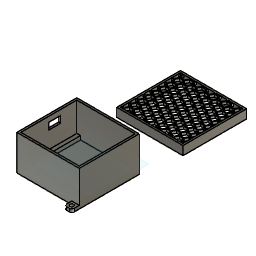
arduino_imu case_ (Autodesk Fusion 360 design; units mm, degrees)
Autodesk Fusion 360 part; units mm, degrees
(part 1 of 2)
sketch "Sketch1" plane through (0, 0, 0) normal (0, 0, 1) x (1, 0, 0)
sketch "Sketch2" plane through (0, 0, 0) normal (0, 0, 1) x (1, 0, 0)
  line L0 (0, 0) -> (46.5, 0)
  line L1 (46.5, 0) -> (46.5, 44.5)
  line L2 (46.5, 44.5) -> (0, 44.5)
  line L3 (0, 44.5) -> (0, 0)
  dimension "d1" = 46.5
  dimension "d2" = 44.5
  constraint horizontal L0
  constraint vertical L1
  constraint horizontal L2
  constraint vertical L3
  constraint coincident L0.start L3.end
  measures "d1" distance of L0.start L0.end
  measures "d2" distance of L0.start L2.end
extrude "Extrude1" add sketch "Sketch2" along normal blind 2 makes body 1
sketch "Sketch3" plane through (0, 0, 2) normal (0, 0, 1) x (-1, 0, 0)
  line L0 (0, -44.5) -> (0, 0)
  line L1 (0, 0) -> (-46.5, 0)
  line L2 (-46.5, 0) -> (-46.5, -44.5)
  line L3 (-46.5, -44.5) -> (0, -44.5)
sketch "Sketch4" plane through (0, 0, 2) normal (0, 0, 1) x (-1, 0, 0)
  line L0 (0, -44.5) -> (0, 0)
  line L1 (0, 0) -> (-46.5, 0)
  line L2 (-46.5, 0) -> (-46.5, -44.5)
  line L3 (-46.5, -44.5) -> (0, -44.5)
  line L4 (1.6, 1.6) -> (-48.1, 1.6)
  line L5 (-48.1, 1.6) -> (-48.1, -46.1)
  line L6 (-48.1, -46.1) -> (1.6, -46.1)
  line L7 (1.6, -46.1) -> (1.6, 1.6)
  dimension "d5" = 1.6
extrude "Extrude2" add sketch "Sketch4" against normal blind 22 bodies 1
copy_body "Body->Comp1" bodies 1 removing the originals makes body 2 in component "Component"
sketch "Sketch5" plane through (0, 0, 2.4305) normal (0, 0, 1) x (-1, 0, 0)
  line L0 (0, -33.8) -> (0, 10.7)
  line L1 (0, 10.7) -> (-46.5, 10.7)
  line L2 (-46.5, 10.7) -> (-46.5, -33.8)
  line L3 (-46.5, -33.8) -> (0, -33.8)
  line L4 (0, -33.8) -> (-3, -33.8)
  line L5 (-3, -33.8) -> (-3, 10.7)
  line L6 (-3, 10.7) -> (0, 10.7)
  line L7 (0, 10.7) -> (0, -33.8)
  line L8 (-46.5, -33.8) -> (-43.5, -33.8)
  line L9 (-43.5, -33.8) -> (-43.5, 10.7)
  line L10 (-43.5, 10.7) -> (-46.5, 10.7)
  line L11 (-46.5, 10.7) -> (-46.5, -33.8)
  dimension "d8" = 3
  dimension "d9" = 3
  constraint horizontal L4
  constraint vertical L5
  constraint horizontal L6
  constraint vertical L7
  constraint coincident L1 L5.end
  constraint coincident L0.start L3.end
  constraint horizontal L8
  constraint vertical L9
  constraint horizontal L10
  constraint vertical L11
  constraint coincident L1 L9.end
  constraint coincident L2.end L3.start
  measures "d8" distance of L0.start L4.end
  measures "d9" distance of L2.end L8.end
extrude "Extrude1'" add sketch "Sketch5" along normal blind 3 contours L0 L1 L3 L4 L5 L6 L7 | L1 L2 L3 L8 L9 L10 L11 sketch seen with x (1, 0, 0) y (0, -1, 0) z (0, 0, -1) at (0, 33.8, 2.4305) bodies 2 in component "Component"
sketch "Sketch6" plane through (0, 0, 0) normal (1, 0, 0) x (0, 1, 0)
  line L0 (-10.7, 5.4305) -> (33.8, 5.4305)
  line L1 (33.8, 5.4305) -> (33.8, 22.4305)
  line L2 (33.8, 22.4305) -> (-10.7, 22.4305)
  line L3 (-10.7, 22.4305) -> (-10.7, 5.4305)
  line L4 (11.55, 5.4305) -> (11.55, 20.4305)
  line L5 (16.55, 17.9305) -> (6.55, 17.9305)
  line L6 (6.55, 17.9305) -> (6.55, 22.9305)
  line L7 (6.55, 22.9305) -> (16.55, 22.9305)
  line L8 (16.55, 22.9305) -> (16.55, 17.9305)
  line L9 (16.55, 17.9305) -> (6.55, 22.9305) construction
  line L10 (6.55, 17.9305) -> (16.55, 22.9305) construction
  point P0 (11.55, 20.4305)
  dimension "d12" = 15
  dimension "d13" = 10
  dimension "d14" = 5
  constraint midpoint L0 L4.start
  constraint perpendicular L0 L4
  constraint horizontal L5
  constraint perpendicular L5 L6
  constraint parallel L5 L7
  constraint parallel L6 L8
  constraint coincident L9 P0
  constraint coincident L10 P0
  constraint coincident P0 L4.end
  measures "d12" distance of L4.start P0
  measures "d13" distance of L6.end L7.end
  measures "d14" distance of L5.end L6.end
extrude "Extrude2'" add 1 faces at (31, 45.5667, -20) along direction (0, 0, -1) blind 2 on bodies 2 bodies 2 in component "Component"
extrude "Extrude3" cut sketch "Sketch6" against normal blind 2.5 contours L2 L5 L6 L8 | L2 L6 L7 L8 sketch seen with x (1, 0, 0) y (0, -1, 0) z (0, 0, -1) at (0, 33.8, 2.4305) bodies 2 in component "Component"
sketch "Sketch7" plane through (0, 0, 24.4305) normal (0, 0, 1) x (-1, 0, 0)
  line L0 (-46.5, 10.7) -> (0, 10.7)
  line L1 (0, 10.7) -> (0, -33.8)
  line L2 (0, -33.8) -> (-46.5, -33.8)
  line L3 (-46.5, -33.8) -> (-46.5, 10.7)
  line L4 (1.6, -35.4) -> (1.6, 12.3)
  line L5 (1.6, 12.3) -> (-48.1, 12.3)
  line L6 (-48.1, 12.3) -> (-48.1, -35.4)
  line L7 (-48.1, -35.4) -> (1.6, -35.4)
  line L8 (0, 10.7) -> (-46.5, 10.7)
  line L9 (-46.5, 10.7) -> (-46.5, -33.8)
  line L10 (-46.5, -33.8) -> (0, -33.8)
  line L11 (0, -33.8) -> (0, 10.7)
  line L12 (0, -33.8) -> (-46.5, -33.8)
  line L13 (0, 10.7) -> (0, -33.8)
  line L14 (-46.5, 10.7) -> (0, 10.7)
  line L15 (-46.5, -33.8) -> (-46.5, 10.7)
  line L16 (-1, 9.7) -> (-45.5, 9.7)
  line L17 (-45.5, 9.7) -> (-45.5, -32.8)
  line L18 (-45.5, -32.8) -> (-1, -32.8)
  line L19 (-1, -32.8) -> (-1, 9.7)
  dimension "d19" = -1
  constraint horizontal L8
  constraint vertical L9
  constraint horizontal L10
  constraint vertical L11
  constraint coincident L2.end L3.start
  constraint coincident L0.end L1.start
extrude "Extrude1''" add sketch "Sketch7" against normal blind 3 separate body contours L0 L1 L2 L3 L8 L9 L10 L11 L12 L13 L14 L15 makes body 3 in component "Component'"
sketch "Sketch8" plane through (0, 0, 24.4305) normal (0, 0, 1) x (-1, 0, 0)
  line L0 (-1, 9.7) -> (-1, -32.8)
  line L1 (-1, -32.8) -> (-45.5, -32.8)
  line L2 (-45.5, -32.8) -> (-45.5, 9.7)
  line L3 (-45.5, 9.7) -> (-1, 9.7)
  line L4 (-46.5, -33.8) -> (0, -33.8)
  line L5 (0, -33.8) -> (0, 10.7)
  line L6 (0, 10.7) -> (-46.5, 10.7)
  line L7 (-46.5, 10.7) -> (-46.5, -33.8)
  line L8 (1, 1) -> (-48, 1)
  line L9 (-48, 1) -> (-48, -35)
  line L10 (-48, -35) -> (1, -35)
  line L11 (1, -35) -> (1, 1)
  constraint horizontal L8
  constraint vertical L9
  constraint horizontal L10
  constraint vertical L11
extrude "Extrude2''" add sketch "Sketch8" along normal blind 1.5 contours L0 L1 L2 L4 L5 L7 L8 | L0 L1 L2 L8 | L4 L5 L7 L8 L9 L10 L11 bodies 3 in component "Component'"
move_body "Move1" bodies 3 to x (1, 0, 0) y (0, -1, 0) z (0, 0, -1) at (-0.0377, 29.218, 33.0505) in component "Component'"
sketch "Sketch9" plane through (0, 0, 2.2652) normal (0, 0, 1) x (-1, 0, 0)
  line L0 (-2.9332, -33.7586) -> (-2.9332, 10.7414)
  line L1 (-2.9332, 10.7414) -> (-43.4332, 10.7414)
  line L2 (-43.4332, 10.7414) -> (-43.4332, -33.7586)
  line L3 (-43.4332, -33.7586) -> (-2.9332, -33.7586)
sketch "Sketch10" plane through (0, 0, 2.2652) normal (0, 0, 1) x (-1, 0, 0)
  line L0 (-43.4332, -33.7586) -> (-2.9332, -33.7586)
  line L1 (-2.9332, -33.7586) -> (-2.9332, 10.7414)
  circle A0 centre (-14.9332, 8.7414) radius 2.5
  point P0 (-14.9332, 8.7414)
  dimension "d24" = 42.5
  dimension "d25" = 12
  dimension "d52" = 5
  constraint coincident P0 A0.centre
  measures "d24" distance of P0 L0
  measures "d25" distance of P0 L1
  measures "d52" diameter of A0
extrude "Extrude4" add sketch "Sketch10" along normal blind 17 sketch seen with x (1, 0, 0) y (0, -1, 0) z (0, 0, -1) at (0.0668, 33.7586, 2.2652) bodies 2 in component "Component"
hole "Hole1" at (15.0254, 42.4284, -17) direction (0, 0, 1) diameter 3.1 depth 6 tip angle 118 bodies 2 in component "Component"
extrude "Extrude5" cut 1 faces at (-1.0667, 17.25, -17.1667) along direction (0, -1, 0) blind 5 on bodies 2 bodies 2 in component "Component"
extrude "Extrude6" add 1 faces at (-0.5333, 27.25, -17.1667) along direction (0, -1, 0) blind 5 on bodies 2 bodies 2 in component "Component"
extrude "Extrude7" add 1 faces at (31, 45.5667, -22) along direction (0, 0, -1) blind 2 on bodies 2 bodies 2 in component "Component"
extrude "Extrude8" add 1 faces at (-1.0667, 15.5833, -15.5) along direction (0, 0, -1) blind 2 on bodies 2 bodies 2 in component "Component"
extrude "Extrude9" cut 1 faces at (-1.0667, 15.5833, -20.5) along direction (0, 0, -1) blind 2.3 on bodies 2 bodies 2 in component "Component"
sketch "Sketch11" plane through (0, 0, 5.2652) normal (0, 0, 1) x (-1, 0, 0)
  line L0 (-46.4332, 10.7414) -> (-46.4332, -33.7586)
  line L1 (-46.4332, -33.7586) -> (-43.4332, -33.7586)
  line L2 (-43.4332, -33.7586) -> (-43.4332, 10.7414)
  line L3 (-43.4332, 10.7414) -> (-46.4332, 10.7414)
  line L4 (-46.4332, -0.2586) -> (-43.4332, -0.2586)
  line L5 (-43.4332, -0.2586) -> (-43.4332, 1.4358)
  line L6 (-43.4332, 1.4358) -> (-46.4332, 1.4358)
  line L7 (-46.4332, 1.4358) -> (-46.4332, -0.2586)
  dimension "d41" = 33.5
  constraint horizontal L4
  constraint vertical L5
  constraint horizontal L6
  constraint vertical L7
  constraint coincident L2 L5.end
  constraint coincident L0 L4.start
  measures "d41" distance of L1 L4
extrude "Extrude10" add sketch "Sketch11" along normal blind 2 contours L0 L2 L4 L5 L6 L7 sketch seen with x (1, 0, 0) y (0, -1, 0) z (0, 0, -1) at (0.0668, 33.7586, 2.2652) bodies 2 in component "Component"
ref_plane "WorkPlane1" through (23.1832, 11.5086, 13.2652) normal (1, 0, 0) x (0, 1, 0)
mirror "Mirror1" about plane through (23.25, 22.25, -11) normal (1, 0, 0) of "Extrude10" in component "Component"
extrude "Extrude11" add 1 faces at (-1.0667, 15.5833, -22.8) along direction (0, 0, 1) blind 1 on bodies 2 bodies 2 in component "Component"
extrude "Extrude12" cut 1 faces at (-1.0667, 15.5833, -17.5) along direction (0, 0, 1) blind 1 on bodies 2 bodies 2 in component "Component"
extrude "Extrude13" add 1 faces at (-1.0667, 12.25, -18.2667) along direction (0, 1, 0) blind 0.5 on bodies 2 bodies 2 in component "Component"
extrude "Extrude14" add 1 faces at (31, 45.5667, -24) along direction (0, 0, -1) blind 2 on bodies 2 bodies 2 in component "Component"
sketch "Sketch12" plane through (0, -12.3414, 0) normal (0, -1, 0) x (1, 0, 0)
  line L0 (-1.6668, 0.2652) -> (48.0332, 0.2652)
  line L1 (48.0332, 0.2652) -> (48.0332, 28.2652)
  line L2 (48.0332, 28.2652) -> (-1.6668, 28.2652)
  line L3 (-1.6668, 28.2652) -> (-1.6668, 0.2652)
  line L4 (48.0332, 0.2652) -> (42.0332, 0.2652)
  line L5 (42.0332, 0.2652) -> (42.0332, 2.7652)
  line L6 (42.0332, 2.7652) -> (48.0332, 2.7652)
  line L7 (48.0332, 2.7652) -> (48.0332, 0.2652)
  dimension "d55" = 6
  dimension "d56" = 2.5
  constraint horizontal L4
  constraint vertical L5
  constraint horizontal L6
  constraint vertical L7
  constraint coincident L0.end L1.start
  measures "d55" distance of L0.end L4.end
  measures "d56" distance of L0.end L6.end
extrude "Extrude15" add sketch "Sketch12" along normal blind 6 contours L0 L1 L4 L5 L6 L7 sketch seen with x (1, 0, 0) y (0, -1, 0) z (0, 0, -1) at (0.0668, 33.7586, 2.2652) bodies 2 in component "Component"
hole "Hole2" at (45.1, 49.1, -0.5) direction (0, 0, 1) diameter 3 depth 7 tip angle 118 bodies 2 in component "Component"
sketch "Sketch13" plane through (0, 35.3586, 0) normal (0, 1, 0) x (-1, 0, 0)
  line L0 (-48.0332, 0.2652) -> (1.6668, 0.2652)
  line L1 (1.6668, 0.2652) -> (1.6668, 28.2652)
  line L2 (1.6668, 28.2652) -> (-48.0332, 28.2652)
  line L3 (-48.0332, 28.2652) -> (-48.0332, 0.2652)
  line L4 (1.6668, 0.2652) -> (-4.3332, 0.2652)
  line L5 (-4.3332, 0.2652) -> (-4.3332, 2.7652)
  line L6 (-4.3332, 2.7652) -> (1.6668, 2.7652)
  line L7 (1.6668, 2.7652) -> (1.6668, 0.2652)
  dimension "d62" = 6
  dimension "d63" = 2.5
  constraint horizontal L4
  constraint vertical L5
  constraint horizontal L6
  constraint vertical L7
  constraint coincident L0.end L1.start
  measures "d62" distance of L0.end L4.end
  measures "d63" distance of L0.end L6.end
extrude "Extrude16" add sketch "Sketch13" along normal blind 6 contours L0 L1 L4 L5 L6 L7 sketch seen with x (1, 0, 0) y (0, -1, 0) z (0, 0, -1) at (0.0668, 33.7586, 2.2652) bodies 2 in component "Component"
hole "Hole3" at (1.4, -4.6, -0.5) direction (0, 0, 1) diameter 3 depth 7 tip angle 118 bodies 2 in component "Component"
fillet "Fillet1" radius 2 4 edges at (48.1, 52.1, 0.75) (42.1, 52.1, 0.75) (4.4, -7.6, 0.75) (-1.6, -7.6, 0.75) on bodies 2 in component "Component"
sketch "Sketch14" plane through (0, 0, 28.2652) normal (0, 0, 1) x (-1, 0, 0)
  line L0 (-46.4332, 10.7414) -> (0.0668, 10.7414)
  line L1 (0.0668, 10.7414) -> (0.0668, -33.7586)
  line L2 (0.0668, -33.7586) -> (-46.4332, -33.7586)
  line L3 (-46.4332, -33.7586) -> (-46.4332, 10.7414)
  line L4 (1.6668, -35.3586) -> (1.6668, 12.3414)
  line L5 (1.6668, 12.3414) -> (-48.0332, 12.3414)
  line L6 (-48.0332, 12.3414) -> (-48.0332, -35.3586)
  line L7 (-48.0332, -35.3586) -> (1.6668, -35.3586)
  line L8 (-49.5332, -36.8586) -> (3.1668, -36.8586)
  line L9 (3.1668, -36.8586) -> (3.1668, 13.8414)
  line L10 (3.1668, 13.8414) -> (-49.5332, 13.8414)
  line L11 (-49.5332, 13.8414) -> (-49.5332, -36.8586)
  dimension "d71" = 1.5
extrude "Extrude1'''" add sketch "Sketch14" against normal blind 4 separate body contours L8 L9 L10 L11 makes body 4 in component "Component''"
sketch "Sketch15" plane through (0, 0, 28.2652) normal (0, 0, 1) x (-1, 0, 0)
  line L0 (1.6668, -35.3586) -> (-48.0332, -35.3586)
  line L1 (-48.0332, -35.3586) -> (-48.0332, 12.3414)
  line L2 (-48.0332, 12.3414) -> (1.6668, 12.3414)
  line L3 (1.6668, 12.3414) -> (1.6668, -35.3586)
  line L4 (-49.5332, 13.8414) -> (-49.5332, -36.8586)
  line L5 (-49.5332, -36.8586) -> (3.1668, -36.8586)
  line L6 (3.1668, -36.8586) -> (3.1668, 13.8414)
  line L7 (3.1668, 13.8414) -> (-49.5332, 13.8414)
extrude "Extrude2'''" add sketch "Sketch15" along normal blind 2 contours L0 L1 L2 L3 | L4 L5 L6 L7 bodies 4 in component "Component''"
sketch "Sketch16" plane through (0, 0, 6.5217) normal (0, 0, -1) x (1, 0, 0)
  line L0 (51.3034, -114.6661) -> (51.3034, -66.9661)
  line L1 (51.3034, -66.9661) -> (1.6034, -66.9661)
  line L2 (1.6034, -66.9661) -> (1.6034, -114.6661)
  line L3 (1.6034, -114.6661) -> (51.3034, -114.6661)
  line L4 (51.3034, -90.8161) -> (1.6034, -90.8161)
  line L5 (26.4534, -114.6661) -> (26.4534, -90.8161)
  line L6 (27.8967, -93.3161) -> (29.3401, -90.8161)
  line L7 (29.3401, -90.8161) -> (27.8967, -88.3161)
  line L8 (27.8967, -88.3161) -> (25.01, -88.3161)
  line L9 (25.01, -88.3161) -> (23.5666, -90.8161)
  line L10 (23.5666, -90.8161) -> (25.01, -93.3161)
  line L11 (25.01, -93.3161) -> (27.8967, -93.3161)
  line L12 (28.6184, -89.5661) -> (26.4534, -90.8161)
  line L13 (24.2883, -89.5661) -> (26.4534, -90.8161)
  line L14 (26.4534, -90.8161) -> (28.6184, -92.0661)
  line L15 (26.4534, -90.8161) -> (24.2883, -92.0661)
  line L16 (26.4534, -90.8161) -> (26.4534, -93.3161)
  line L17 (26.4534, -90.8161) -> (26.4534, -88.3161)
  line L18 (-41.3853, -93.3161) -> (-39.9419, -90.8161)
  line L19 (-44.272, -93.3161) -> (-41.3853, -93.3161)
  line L20 (-45.7154, -90.8161) -> (-44.272, -93.3161)
  line L21 (-44.272, -88.3161) -> (-45.7154, -90.8161)
  line L22 (-41.3853, -88.3161) -> (-44.272, -88.3161)
  line L23 (-39.9419, -90.8161) -> (-41.3853, -88.3161)
  line L24 (-36.4366, -96.1733) -> (-34.9932, -93.6733)
  line L25 (-39.3233, -96.1733) -> (-36.4366, -96.1733)
  line L26 (-40.7667, -93.6733) -> (-39.3233, -96.1733)
  line L27 (-39.3233, -91.1733) -> (-40.7667, -93.6733)
  line L28 (-36.4366, -91.1733) -> (-39.3233, -91.1733)
  line L29 (-34.9932, -93.6733) -> (-36.4366, -91.1733)
  line L30 (-31.4879, -99.0304) -> (-30.0445, -96.5304)
  line L31 (-34.3746, -99.0304) -> (-31.4879, -99.0304)
  line L32 (-35.818, -96.5304) -> (-34.3746, -99.0304)
  line L33 (-34.3746, -94.0304) -> (-35.818, -96.5304)
  line L34 (-31.4879, -94.0304) -> (-34.3746, -94.0304)
  line L35 (-30.0445, -96.5304) -> (-31.4879, -94.0304)
  line L36 (-26.5391, -101.8875) -> (-25.0958, -99.3875)
  line L37 (-29.4259, -101.8875) -> (-26.5391, -101.8875)
  line L38 (-30.8693, -99.3875) -> (-29.4259, -101.8875)
  line L39 (-29.4259, -96.8875) -> (-30.8693, -99.3875)
  line L40 (-26.5391, -96.8875) -> (-29.4259, -96.8875)
  line L41 (-25.0958, -99.3875) -> (-26.5391, -96.8875)
  line L42 (-21.5904, -104.7447) -> (-20.147, -102.2447)
  line L43 (-24.4772, -104.7447) -> (-21.5904, -104.7447)
  line L44 (-25.9205, -102.2447) -> (-24.4772, -104.7447)
  line L45 (-24.4772, -99.7447) -> (-25.9205, -102.2447)
  line L46 (-21.5904, -99.7447) -> (-24.4772, -99.7447)
  line L47 (-20.147, -102.2447) -> (-21.5904, -99.7447)
  line L48 (-16.6417, -107.6018) -> (-15.1983, -105.1018)
  line L49 (-19.5285, -107.6018) -> (-16.6417, -107.6018)
  line L50 (-20.9718, -105.1018) -> (-19.5285, -107.6018)
  line L51 (-19.5285, -102.6018) -> (-20.9718, -105.1018)
  line L52 (-16.6417, -102.6018) -> (-19.5285, -102.6018)
  line L53 (-15.1983, -105.1018) -> (-16.6417, -102.6018)
  line L54 (-11.693, -110.459) -> (-10.2496, -107.959)
  line L55 (-14.5797, -110.459) -> (-11.693, -110.459)
  line L56 (-16.0231, -107.959) -> (-14.5797, -110.459)
  line L57 (-14.5797, -105.459) -> (-16.0231, -107.959)
  line L58 (-11.693, -105.459) -> (-14.5797, -105.459)
  line L59 (-10.2496, -107.959) -> (-11.693, -105.459)
  line L60 (-6.7443, -113.3161) -> (-5.3009, -110.8161)
  line L61 (-9.631, -113.3161) -> (-6.7443, -113.3161)
  line L62 (-11.0744, -110.8161) -> (-9.631, -113.3161)
  line L63 (-9.631, -108.3161) -> (-11.0744, -110.8161)
  line L64 (-6.7443, -108.3161) -> (-9.631, -108.3161)
  line L65 (-5.3009, -110.8161) -> (-6.7443, -108.3161)
  line L66 (-1.7956, -116.1733) -> (-0.3522, -113.6733)
  line L67 (-4.6823, -116.1733) -> (-1.7956, -116.1733)
  line L68 (-6.1257, -113.6733) -> (-4.6823, -116.1733)
  line L69 (-4.6823, -111.1733) -> (-6.1257, -113.6733)
  line L70 (-1.7956, -111.1733) -> (-4.6823, -111.1733)
  line L71 (-0.3522, -113.6733) -> (-1.7956, -111.1733)
  line L72 (3.1532, -119.0304) -> (4.5965, -116.5304)
  line L73 (0.2664, -119.0304) -> (3.1532, -119.0304)
  line L74 (-1.177, -116.5304) -> (0.2664, -119.0304)
  line L75 (0.2664, -114.0304) -> (-1.177, -116.5304)
  line L76 (3.1532, -114.0304) -> (0.2664, -114.0304)
  line L77 (4.5965, -116.5304) -> (3.1532, -114.0304)
  line L78 (8.1019, -121.8875) -> (9.5453, -119.3875)
  line L79 (5.2151, -121.8875) -> (8.1019, -121.8875)
  line L80 (3.7718, -119.3875) -> (5.2151, -121.8875)
  line L81 (5.2151, -116.8875) -> (3.7718, -119.3875)
  line L82 (8.1019, -116.8875) -> (5.2151, -116.8875)
  line L83 (9.5453, -119.3875) -> (8.1019, -116.8875)
  line L84 (13.0506, -124.7447) -> (14.494, -122.2447)
  line L85 (10.1638, -124.7447) -> (13.0506, -124.7447)
  line L86 (8.7205, -122.2447) -> (10.1638, -124.7447)
  line L87 (10.1638, -119.7447) -> (8.7205, -122.2447)
  line L88 (13.0506, -119.7447) -> (10.1638, -119.7447)
  line L89 (14.494, -122.2447) -> (13.0506, -119.7447)
  line L90 (17.9993, -127.6018) -> (19.4427, -125.1018)
  line L91 (15.1126, -127.6018) -> (17.9993, -127.6018)
  line L92 (13.6692, -125.1018) -> (15.1126, -127.6018)
  line L93 (15.1126, -122.6018) -> (13.6692, -125.1018)
  line L94 (17.9993, -122.6018) -> (15.1126, -122.6018)
  line L95 (19.4427, -125.1018) -> (17.9993, -122.6018)
  line L96 (22.948, -130.459) -> (24.3914, -127.959)
  line L97 (20.0613, -130.459) -> (22.948, -130.459)
  line L98 (18.6179, -127.959) -> (20.0613, -130.459)
  line L99 (20.0613, -125.459) -> (18.6179, -127.959)
  line L100 (22.948, -125.459) -> (20.0613, -125.459)
  line L101 (24.3914, -127.959) -> (22.948, -125.459)
  line L102 (27.8967, -133.3161) -> (29.3401, -130.8161)
  line L103 (25.01, -133.3161) -> (27.8967, -133.3161)
  line L104 (23.5666, -130.8161) -> (25.01, -133.3161)
  line L105 (25.01, -128.3161) -> (23.5666, -130.8161)
  line L106 (27.8967, -128.3161) -> (25.01, -128.3161)
  line L107 (29.3401, -130.8161) -> (27.8967, -128.3161)
  line L108 (-36.4366, -90.459) -> (-34.9932, -87.959)
  line L109 (-39.3233, -90.459) -> (-36.4366, -90.459)
  line L110 (-40.7667, -87.959) -> (-39.3233, -90.459)
  line L111 (-39.3233, -85.459) -> (-40.7667, -87.959)
  line L112 (-36.4366, -85.459) -> (-39.3233, -85.459)
  line L113 (-34.9932, -87.959) -> (-36.4366, -85.459)
  line L114 (-31.4879, -93.3161) -> (-30.0445, -90.8161)
  line L115 (-34.3746, -93.3161) -> (-31.4879, -93.3161)
  line L116 (-35.818, -90.8161) -> (-34.3746, -93.3161)
  line L117 (-34.3746, -88.3161) -> (-35.818, -90.8161)
  line L118 (-31.4879, -88.3161) -> (-34.3746, -88.3161)
  line L119 (-30.0445, -90.8161) -> (-31.4879, -88.3161)
  line L120 (-26.5391, -96.1733) -> (-25.0958, -93.6733)
  line L121 (-29.4259, -96.1733) -> (-26.5391, -96.1733)
  line L122 (-30.8693, -93.6733) -> (-29.4259, -96.1733)
  line L123 (-29.4259, -91.1733) -> (-30.8693, -93.6733)
  line L124 (-26.5391, -91.1733) -> (-29.4259, -91.1733)
  line L125 (-25.0958, -93.6733) -> (-26.5391, -91.1733)
  line L126 (-21.5904, -99.0304) -> (-20.147, -96.5304)
  line L127 (-24.4772, -99.0304) -> (-21.5904, -99.0304)
  line L128 (-25.9205, -96.5304) -> (-24.4772, -99.0304)
  line L129 (-24.4772, -94.0304) -> (-25.9205, -96.5304)
  line L130 (-21.5904, -94.0304) -> (-24.4772, -94.0304)
  line L131 (-20.147, -96.5304) -> (-21.5904, -94.0304)
  line L132 (-16.6417, -101.8875) -> (-15.1983, -99.3875)
  line L133 (-19.5285, -101.8875) -> (-16.6417, -101.8875)
  line L134 (-20.9718, -99.3875) -> (-19.5285, -101.8875)
  line L135 (-19.5285, -96.8875) -> (-20.9718, -99.3875)
  line L136 (-16.6417, -96.8875) -> (-19.5285, -96.8875)
  line L137 (-15.1983, -99.3875) -> (-16.6417, -96.8875)
  line L138 (-11.693, -104.7447) -> (-10.2496, -102.2447)
  line L139 (-14.5797, -104.7447) -> (-11.693, -104.7447)
  line L140 (-16.0231, -102.2447) -> (-14.5797, -104.7447)
  line L141 (-14.5797, -99.7447) -> (-16.0231, -102.2447)
  line L142 (-11.693, -99.7447) -> (-14.5797, -99.7447)
  line L143 (-10.2496, -102.2447) -> (-11.693, -99.7447)
  line L144 (-6.7443, -107.6018) -> (-5.3009, -105.1018)
  line L145 (-9.631, -107.6018) -> (-6.7443, -107.6018)
  line L146 (-11.0744, -105.1018) -> (-9.631, -107.6018)
  line L147 (-9.631, -102.6018) -> (-11.0744, -105.1018)
  line L148 (-6.7443, -102.6018) -> (-9.631, -102.6018)
  line L149 (-5.3009, -105.1018) -> (-6.7443, -102.6018)
  line L150 (-1.7956, -110.459) -> (-0.3522, -107.959)
  line L151 (-4.6823, -110.459) -> (-1.7956, -110.459)
  line L152 (-6.1257, -107.959) -> (-4.6823, -110.459)
  line L153 (-4.6823, -105.459) -> (-6.1257, -107.959)
  line L154 (-1.7956, -105.459) -> (-4.6823, -105.459)
  line L155 (-0.3522, -107.959) -> (-1.7956, -105.459)
  line L156 (3.1532, -113.3161) -> (4.5965, -110.8161)
  line L157 (0.2664, -113.3161) -> (3.1532, -113.3161)
  line L158 (-1.177, -110.8161) -> (0.2664, -113.3161)
  line L159 (0.2664, -108.3161) -> (-1.177, -110.8161)
  line L160 (3.1532, -108.3161) -> (0.2664, -108.3161)
  line L161 (4.5965, -110.8161) -> (3.1532, -108.3161)
  line L162 (8.1019, -116.1733) -> (9.5453, -113.6733)
  line L163 (5.2151, -116.1733) -> (8.1019, -116.1733)
  line L164 (3.7718, -113.6733) -> (5.2151, -116.1733)
  line L165 (5.2151, -111.1733) -> (3.7718, -113.6733)
  line L166 (8.1019, -111.1733) -> (5.2151, -111.1733)
  line L167 (9.5453, -113.6733) -> (8.1019, -111.1733)
  line L168 (13.0506, -119.0304) -> (14.494, -116.5304)
  line L169 (10.1638, -119.0304) -> (13.0506, -119.0304)
  line L170 (8.7205, -116.5304) -> (10.1638, -119.0304)
  line L171 (10.1638, -114.0304) -> (8.7205, -116.5304)
  line L172 (13.0506, -114.0304) -> (10.1638, -114.0304)
  line L173 (14.494, -116.5304) -> (13.0506, -114.0304)
  line L174 (17.9993, -121.8875) -> (19.4427, -119.3875)
  line L175 (15.1126, -121.8875) -> (17.9993, -121.8875)
  line L176 (13.6692, -119.3875) -> (15.1126, -121.8875)
  line L177 (15.1126, -116.8875) -> (13.6692, -119.3875)
  line L178 (17.9993, -116.8875) -> (15.1126, -116.8875)
  line L179 (19.4427, -119.3875) -> (17.9993, -116.8875)
  line L180 (22.948, -124.7447) -> (24.3914, -122.2447)
  line L181 (20.0613, -124.7447) -> (22.948, -124.7447)
  line L182 (18.6179, -122.2447) -> (20.0613, -124.7447)
  line L183 (20.0613, -119.7447) -> (18.6179, -122.2447)
  line L184 (22.948, -119.7447) -> (20.0613, -119.7447)
  line L185 (24.3914, -122.2447) -> (22.948, -119.7447)
  line L186 (27.8967, -127.6018) -> (29.3401, -125.1018)
  line L187 (25.01, -127.6018) -> (27.8967, -127.6018)
  line L188 (23.5666, -125.1018) -> (25.01, -127.6018)
  line L189 (25.01, -122.6018) -> (23.5666, -125.1018)
  line L190 (27.8967, -122.6018) -> (25.01, -122.6018)
  line L191 (29.3401, -125.1018) -> (27.8967, -122.6018)
  line L192 (32.8455, -130.459) -> (34.2888, -127.959)
  line L193 (29.9587, -130.459) -> (32.8455, -130.459)
  line L194 (28.5153, -127.959) -> (29.9587, -130.459)
  line L195 (29.9587, -125.459) -> (28.5153, -127.959)
  line L196 (32.8455, -125.459) -> (29.9587, -125.459)
  line L197 (34.2888, -127.959) -> (32.8455, -125.459)
  line L198 (-31.4879, -87.6018) -> (-30.0445, -85.1018)
  line L199 (-34.3746, -87.6018) -> (-31.4879, -87.6018)
  line L200 (-35.818, -85.1018) -> (-34.3746, -87.6018)
  line L201 (-34.3746, -82.6018) -> (-35.818, -85.1018)
  line L202 (-31.4879, -82.6018) -> (-34.3746, -82.6018)
  line L203 (-30.0445, -85.1018) -> (-31.4879, -82.6018)
  line L204 (-26.5391, -90.459) -> (-25.0958, -87.959)
  line L205 (-29.4259, -90.459) -> (-26.5391, -90.459)
  line L206 (-30.8693, -87.959) -> (-29.4259, -90.459)
  line L207 (-29.4259, -85.459) -> (-30.8693, -87.959)
  line L208 (-26.5391, -85.459) -> (-29.4259, -85.459)
  line L209 (-25.0958, -87.959) -> (-26.5391, -85.459)
  line L210 (-21.5904, -93.3161) -> (-20.147, -90.8161)
  line L211 (-24.4772, -93.3161) -> (-21.5904, -93.3161)
  line L212 (-25.9205, -90.8161) -> (-24.4772, -93.3161)
  line L213 (-24.4772, -88.3161) -> (-25.9205, -90.8161)
  line L214 (-21.5904, -88.3161) -> (-24.4772, -88.3161)
  line L215 (-20.147, -90.8161) -> (-21.5904, -88.3161)
  line L216 (-16.6417, -96.1733) -> (-15.1983, -93.6733)
  line L217 (-19.5285, -96.1733) -> (-16.6417, -96.1733)
  line L218 (-20.9718, -93.6733) -> (-19.5285, -96.1733)
  line L219 (-19.5285, -91.1733) -> (-20.9718, -93.6733)
  line L220 (-16.6417, -91.1733) -> (-19.5285, -91.1733)
  line L221 (-15.1983, -93.6733) -> (-16.6417, -91.1733)
  line L222 (-11.693, -99.0304) -> (-10.2496, -96.5304)
  line L223 (-14.5797, -99.0304) -> (-11.693, -99.0304)
  line L224 (-16.0231, -96.5304) -> (-14.5797, -99.0304)
  line L225 (-14.5797, -94.0304) -> (-16.0231, -96.5304)
  line L226 (-11.693, -94.0304) -> (-14.5797, -94.0304)
  line L227 (-10.2496, -96.5304) -> (-11.693, -94.0304)
  line L228 (-6.7443, -101.8875) -> (-5.3009, -99.3875)
  line L229 (-9.631, -101.8875) -> (-6.7443, -101.8875)
  line L230 (-11.0744, -99.3875) -> (-9.631, -101.8875)
  line L231 (-9.631, -96.8875) -> (-11.0744, -99.3875)
  line L232 (-6.7443, -96.8875) -> (-9.631, -96.8875)
  line L233 (-5.3009, -99.3875) -> (-6.7443, -96.8875)
  line L234 (-1.7956, -104.7447) -> (-0.3522, -102.2447)
  line L235 (-4.6823, -104.7447) -> (-1.7956, -104.7447)
  line L236 (-6.1257, -102.2447) -> (-4.6823, -104.7447)
  line L237 (-4.6823, -99.7447) -> (-6.1257, -102.2447)
  line L238 (-1.7956, -99.7447) -> (-4.6823, -99.7447)
  line L239 (-0.3522, -102.2447) -> (-1.7956, -99.7447)
  line L240 (3.1532, -107.6018) -> (4.5965, -105.1018)
  line L241 (0.2664, -107.6018) -> (3.1532, -107.6018)
  line L242 (-1.177, -105.1018) -> (0.2664, -107.6018)
  line L243 (0.2664, -102.6018) -> (-1.177, -105.1018)
  line L244 (3.1532, -102.6018) -> (0.2664, -102.6018)
  line L245 (4.5965, -105.1018) -> (3.1532, -102.6018)
  line L246 (8.1019, -110.459) -> (9.5453, -107.959)
  line L247 (5.2151, -110.459) -> (8.1019, -110.459)
  line L248 (3.7718, -107.959) -> (5.2151, -110.459)
  line L249 (5.2151, -105.459) -> (3.7718, -107.959)
  line L250 (8.1019, -105.459) -> (5.2151, -105.459)
  line L251 (9.5453, -107.959) -> (8.1019, -105.459)
  line L252 (13.0506, -113.3161) -> (14.494, -110.8161)
  line L253 (10.1638, -113.3161) -> (13.0506, -113.3161)
  line L254 (8.7205, -110.8161) -> (10.1638, -113.3161)
  line L255 (10.1638, -108.3161) -> (8.7205, -110.8161)
  line L256 (13.0506, -108.3161) -> (10.1638, -108.3161)
  line L257 (14.494, -110.8161) -> (13.0506, -108.3161)
  line L258 (17.9993, -116.1733) -> (19.4427, -113.6733)
  line L259 (15.1126, -116.1733) -> (17.9993, -116.1733)
  line L260 (13.6692, -113.6733) -> (15.1126, -116.1733)
  line L261 (15.1126, -111.1733) -> (13.6692, -113.6733)
  line L262 (17.9993, -111.1733) -> (15.1126, -111.1733)
  line L263 (19.4427, -113.6733) -> (17.9993, -111.1733)
  line L264 (22.948, -119.0304) -> (24.3914, -116.5304)
  line L265 (20.0613, -119.0304) -> (22.948, -119.0304)
  line L266 (18.6179, -116.5304) -> (20.0613, -119.0304)
  line L267 (20.0613, -114.0304) -> (18.6179, -116.5304)
  line L268 (22.948, -114.0304) -> (20.0613, -114.0304)
  line L269 (24.3914, -116.5304) -> (22.948, -114.0304)
  line L270 (27.8967, -121.8875) -> (29.3401, -119.3875)
  line L271 (25.01, -121.8875) -> (27.8967, -121.8875)
  line L272 (23.5666, -119.3875) -> (25.01, -121.8875)
  line L273 (25.01, -116.8875) -> (23.5666, -119.3875)
  line L274 (27.8967, -116.8875) -> (25.01, -116.8875)
  line L275 (29.3401, -119.3875) -> (27.8967, -116.8875)
  line L276 (32.8455, -124.7447) -> (34.2888, -122.2447)
  line L277 (29.9587, -124.7447) -> (32.8455, -124.7447)
  line L278 (28.5153, -122.2447) -> (29.9587, -124.7447)
  line L279 (29.9587, -119.7447) -> (28.5153, -122.2447)
  line L280 (32.8455, -119.7447) -> (29.9587, -119.7447)
  line L281 (34.2888, -122.2447) -> (32.8455, -119.7447)
  line L282 (37.7942, -127.6018) -> (39.2376, -125.1018)
  line L283 (34.9074, -127.6018) -> (37.7942, -127.6018)
  line L284 (33.4641, -125.1018) -> (34.9074, -127.6018)
  line L285 (34.9074, -122.6018) -> (33.4641, -125.1018)
  line L286 (37.7942, -122.6018) -> (34.9074, -122.6018)
  line L287 (39.2376, -125.1018) -> (37.7942, -122.6018)
  line L288 (-26.5391, -84.7447) -> (-25.0958, -82.2447)
  line L289 (-29.4259, -84.7447) -> (-26.5391, -84.7447)
  line L290 (-30.8693, -82.2447) -> (-29.4259, -84.7447)
  line L291 (-29.4259, -79.7447) -> (-30.8693, -82.2447)
  line L292 (-26.5391, -79.7447) -> (-29.4259, -79.7447)
  line L293 (-25.0958, -82.2447) -> (-26.5391, -79.7447)
  line L294 (-21.5904, -87.6018) -> (-20.147, -85.1018)
  line L295 (-24.4772, -87.6018) -> (-21.5904, -87.6018)
  line L296 (-25.9205, -85.1018) -> (-24.4772, -87.6018)
  line L297 (-24.4772, -82.6018) -> (-25.9205, -85.1018)
  line L298 (-21.5904, -82.6018) -> (-24.4772, -82.6018)
  line L299 (-20.147, -85.1018) -> (-21.5904, -82.6018)
  line L300 (-16.6417, -90.459) -> (-15.1983, -87.959)
  line L301 (-19.5285, -90.459) -> (-16.6417, -90.459)
  line L302 (-20.9718, -87.959) -> (-19.5285, -90.459)
  line L303 (-19.5285, -85.459) -> (-20.9718, -87.959)
  line L304 (-16.6417, -85.459) -> (-19.5285, -85.459)
  line L305 (-15.1983, -87.959) -> (-16.6417, -85.459)
  line L306 (-11.693, -93.3161) -> (-10.2496, -90.8161)
  line L307 (-14.5797, -93.3161) -> (-11.693, -93.3161)
  line L308 (-16.0231, -90.8161) -> (-14.5797, -93.3161)
  line L309 (-14.5797, -88.3161) -> (-16.0231, -90.8161)
  line L310 (-11.693, -88.3161) -> (-14.5797, -88.3161)
  line L311 (-10.2496, -90.8161) -> (-11.693, -88.3161)
  line L312 (-6.7443, -96.1733) -> (-5.3009, -93.6733)
  line L313 (-9.631, -96.1733) -> (-6.7443, -96.1733)
  line L314 (-11.0744, -93.6733) -> (-9.631, -96.1733)
  line L315 (-9.631, -91.1733) -> (-11.0744, -93.6733)
  line L316 (-6.7443, -91.1733) -> (-9.631, -91.1733)
  line L317 (-5.3009, -93.6733) -> (-6.7443, -91.1733)
  line L318 (-1.7956, -99.0304) -> (-0.3522, -96.5304)
  line L319 (-4.6823, -99.0304) -> (-1.7956, -99.0304)
  line L320 (-6.1257, -96.5304) -> (-4.6823, -99.0304)
  line L321 (-4.6823, -94.0304) -> (-6.1257, -96.5304)
  line L322 (-1.7956, -94.0304) -> (-4.6823, -94.0304)
  line L323 (-0.3522, -96.5304) -> (-1.7956, -94.0304)
  line L324 (3.1532, -101.8875) -> (4.5965, -99.3875)
  line L325 (0.2664, -101.8875) -> (3.1532, -101.8875)
  line L326 (-1.177, -99.3875) -> (0.2664, -101.8875)
  line L327 (0.2664, -96.8875) -> (-1.177, -99.3875)
  line L328 (3.1532, -96.8875) -> (0.2664, -96.8875)
  line L329 (4.5965, -99.3875) -> (3.1532, -96.8875)
  line L330 (8.1019, -104.7447) -> (9.5453, -102.2447)
  line L331 (5.2151, -104.7447) -> (8.1019, -104.7447)
  line L332 (3.7718, -102.2447) -> (5.2151, -104.7447)
  line L333 (5.2151, -99.7447) -> (3.7718, -102.2447)
  line L334 (8.1019, -99.7447) -> (5.2151, -99.7447)
  line L335 (9.5453, -102.2447) -> (8.1019, -99.7447)
  line L336 (13.0506, -107.6018) -> (14.494, -105.1018)
  line L337 (10.1638, -107.6018) -> (13.0506, -107.6018)
  line L338 (8.7205, -105.1018) -> (10.1638, -107.6018)
  line L339 (10.1638, -102.6018) -> (8.7205, -105.1018)
  line L340 (13.0506, -102.6018) -> (10.1638, -102.6018)
  line L341 (14.494, -105.1018) -> (13.0506, -102.6018)
  line L342 (17.9993, -110.459) -> (19.4427, -107.959)
  line L343 (15.1126, -110.459) -> (17.9993, -110.459)
  line L344 (13.6692, -107.959) -> (15.1126, -110.459)
  line L345 (15.1126, -105.459) -> (13.6692, -107.959)
  line L346 (17.9993, -105.459) -> (15.1126, -105.459)
  line L347 (19.4427, -107.959) -> (17.9993, -105.459)
  line L348 (22.948, -113.3161) -> (24.3914, -110.8161)
  line L349 (20.0613, -113.3161) -> (22.948, -113.3161)
  line L350 (18.6179, -110.8161) -> (20.0613, -113.3161)
  line L351 (20.0613, -108.3161) -> (18.6179, -110.8161)
  line L352 (22.948, -108.3161) -> (20.0613, -108.3161)
  line L353 (24.3914, -110.8161) -> (22.948, -108.3161)
  line L354 (27.8967, -116.1733) -> (29.3401, -113.6733)
  line L355 (25.01, -116.1733) -> (27.8967, -116.1733)
  line L356 (23.5666, -113.6733) -> (25.01, -116.1733)
  line L357 (25.01, -111.1733) -> (23.5666, -113.6733)
  line L358 (27.8967, -111.1733) -> (25.01, -111.1733)
  line L359 (29.3401, -113.6733) -> (27.8967, -111.1733)
  line L360 (32.8455, -119.0304) -> (34.2888, -116.5304)
  line L361 (29.9587, -119.0304) -> (32.8455, -119.0304)
  line L362 (28.5153, -116.5304) -> (29.9587, -119.0304)
  line L363 (29.9587, -114.0304) -> (28.5153, -116.5304)
  line L364 (32.8455, -114.0304) -> (29.9587, -114.0304)
  line L365 (34.2888, -116.5304) -> (32.8455, -114.0304)
  line L366 (37.7942, -121.8875) -> (39.2376, -119.3875)
  line L367 (34.9074, -121.8875) -> (37.7942, -121.8875)
  line L368 (33.4641, -119.3875) -> (34.9074, -121.8875)
  line L369 (34.9074, -116.8875) -> (33.4641, -119.3875)
  line L370 (37.7942, -116.8875) -> (34.9074, -116.8875)
  line L371 (39.2376, -119.3875) -> (37.7942, -116.8875)
  line L372 (42.7429, -124.7447) -> (44.1863, -122.2447)
  line L373 (39.8561, -124.7447) -> (42.7429, -124.7447)
  line L374 (38.4128, -122.2447) -> (39.8561, -124.7447)
  line L375 (39.8561, -119.7447) -> (38.4128, -122.2447)
  line L376 (42.7429, -119.7447) -> (39.8561, -119.7447)
  line L377 (44.1863, -122.2447) -> (42.7429, -119.7447)
  line L378 (-21.5904, -81.8875) -> (-20.147, -79.3875)
  line L379 (-24.4772, -81.8875) -> (-21.5904, -81.8875)
  line L380 (-25.9205, -79.3875) -> (-24.4772, -81.8875)
  line L381 (-24.4772, -76.8875) -> (-25.9205, -79.3875)
  line L382 (-21.5904, -76.8875) -> (-24.4772, -76.8875)
  line L383 (-20.147, -79.3875) -> (-21.5904, -76.8875)
  line L384 (-16.6417, -84.7447) -> (-15.1983, -82.2447)
  line L385 (-19.5285, -84.7447) -> (-16.6417, -84.7447)
  line L386 (-20.9718, -82.2447) -> (-19.5285, -84.7447)
  line L387 (-19.5285, -79.7447) -> (-20.9718, -82.2447)
  line L388 (-16.6417, -79.7447) -> (-19.5285, -79.7447)
  line L389 (-15.1983, -82.2447) -> (-16.6417, -79.7447)
  line L390 (-11.693, -87.6018) -> (-10.2496, -85.1018)
  line L391 (-14.5797, -87.6018) -> (-11.693, -87.6018)
  line L392 (-16.0231, -85.1018) -> (-14.5797, -87.6018)
  line L393 (-14.5797, -82.6018) -> (-16.0231, -85.1018)
  line L394 (-11.693, -82.6018) -> (-14.5797, -82.6018)
  line L395 (-10.2496, -85.1018) -> (-11.693, -82.6018)
  line L396 (-6.7443, -90.459) -> (-5.3009, -87.959)
  line L397 (-9.631, -90.459) -> (-6.7443, -90.459)
  line L398 (-11.0744, -87.959) -> (-9.631, -90.459)
  line L399 (-9.631, -85.459) -> (-11.0744, -87.959)
  line L400 (-6.7443, -85.459) -> (-9.631, -85.459)
  line L401 (-5.3009, -87.959) -> (-6.7443, -85.459)
  line L402 (-1.7956, -93.3161) -> (-0.3522, -90.8161)
  line L403 (-4.6823, -93.3161) -> (-1.7956, -93.3161)
  line L404 (-6.1257, -90.8161) -> (-4.6823, -93.3161)
  line L405 (-4.6823, -88.3161) -> (-6.1257, -90.8161)
  line L406 (-1.7956, -88.3161) -> (-4.6823, -88.3161)
  line L407 (-0.3522, -90.8161) -> (-1.7956, -88.3161)
  line L408 (3.1532, -96.1733) -> (4.5965, -93.6733)
  line L409 (0.2664, -96.1733) -> (3.1532, -96.1733)
  line L410 (-1.177, -93.6733) -> (0.2664, -96.1733)
  line L411 (0.2664, -91.1733) -> (-1.177, -93.6733)
  line L412 (3.1532, -91.1733) -> (0.2664, -91.1733)
  line L413 (4.5965, -93.6733) -> (3.1532, -91.1733)
  line L414 (8.1019, -99.0304) -> (9.5453, -96.5304)
  line L415 (5.2151, -99.0304) -> (8.1019, -99.0304)
  line L416 (3.7718, -96.5304) -> (5.2151, -99.0304)
  line L417 (5.2151, -94.0304) -> (3.7718, -96.5304)
  line L418 (8.1019, -94.0304) -> (5.2151, -94.0304)
  line L419 (9.5453, -96.5304) -> (8.1019, -94.0304)
  line L420 (13.0506, -101.8875) -> (14.494, -99.3875)
  line L421 (10.1638, -101.8875) -> (13.0506, -101.8875)
  line L422 (8.7205, -99.3875) -> (10.1638, -101.8875)
  line L423 (10.1638, -96.8875) -> (8.7205, -99.3875)
  line L424 (13.0506, -96.8875) -> (10.1638, -96.8875)
  line L425 (14.494, -99.3875) -> (13.0506, -96.8875)
  line L426 (17.9993, -104.7447) -> (19.4427, -102.2447)
  line L427 (15.1126, -104.7447) -> (17.9993, -104.7447)
  line L428 (13.6692, -102.2447) -> (15.1126, -104.7447)
  line L429 (15.1126, -99.7447) -> (13.6692, -102.2447)
  line L430 (17.9993, -99.7447) -> (15.1126, -99.7447)
  line L431 (19.4427, -102.2447) -> (17.9993, -99.7447)
  line L432 (22.948, -107.6018) -> (24.3914, -105.1018)
  line L433 (20.0613, -107.6018) -> (22.948, -107.6018)
  line L434 (18.6179, -105.1018) -> (20.0613, -107.6018)
  line L435 (20.0613, -102.6018) -> (18.6179, -105.1018)
  line L436 (22.948, -102.6018) -> (20.0613, -102.6018)
  line L437 (24.3914, -105.1018) -> (22.948, -102.6018)
  line L438 (27.8967, -110.459) -> (29.3401, -107.959)
  line L439 (25.01, -110.459) -> (27.8967, -110.459)
  line L440 (23.5666, -107.959) -> (25.01, -110.459)
  line L441 (25.01, -105.459) -> (23.5666, -107.959)
  line L442 (27.8967, -105.459) -> (25.01, -105.459)
  line L443 (29.3401, -107.959) -> (27.8967, -105.459)
  line L444 (32.8455, -113.3161) -> (34.2888, -110.8161)
  line L445 (29.9587, -113.3161) -> (32.8455, -113.3161)
  line L446 (28.5153, -110.8161) -> (29.9587, -113.3161)
  line L447 (29.9587, -108.3161) -> (28.5153, -110.8161)
  line L448 (32.8455, -108.3161) -> (29.9587, -108.3161)
  line L449 (34.2888, -110.8161) -> (32.8455, -108.3161)
  line L450 (37.7942, -116.1733) -> (39.2376, -113.6733)
  line L451 (34.9074, -116.1733) -> (37.7942, -116.1733)
  line L452 (33.4641, -113.6733) -> (34.9074, -116.1733)
  line L453 (34.9074, -111.1733) -> (33.4641, -113.6733)
  line L454 (37.7942, -111.1733) -> (34.9074, -111.1733)
  line L455 (39.2376, -113.6733) -> (37.7942, -111.1733)
  line L456 (42.7429, -119.0304) -> (44.1863, -116.5304)
  line L457 (39.8561, -119.0304) -> (42.7429, -119.0304)
  line L458 (38.4128, -116.5304) -> (39.8561, -119.0304)
  line L459 (39.8561, -114.0304) -> (38.4128, -116.5304)
  line L460 (42.7429, -114.0304) -> (39.8561, -114.0304)
  line L461 (44.1863, -116.5304) -> (42.7429, -114.0304)
  line L462 (47.6916, -121.8875) -> (49.135, -119.3875)
  line L463 (44.8049, -121.8875) -> (47.6916, -121.8875)
  line L464 (43.3615, -119.3875) -> (44.8049, -121.8875)
  line L465 (44.8049, -116.8875) -> (43.3615, -119.3875)
  line L466 (47.6916, -116.8875) -> (44.8049, -116.8875)
  line L467 (49.135, -119.3875) -> (47.6916, -116.8875)
  line L468 (-16.6417, -79.0304) -> (-15.1983, -76.5304)
  line L469 (-19.5285, -79.0304) -> (-16.6417, -79.0304)
  line L470 (-20.9718, -76.5304) -> (-19.5285, -79.0304)
  line L471 (-19.5285, -74.0304) -> (-20.9718, -76.5304)
  line L472 (-16.6417, -74.0304) -> (-19.5285, -74.0304)
  line L473 (-15.1983, -76.5304) -> (-16.6417, -74.0304)
  line L474 (-11.693, -81.8875) -> (-10.2496, -79.3875)
  line L475 (-14.5797, -81.8875) -> (-11.693, -81.8875)
  line L476 (-16.0231, -79.3875) -> (-14.5797, -81.8875)
  line L477 (-14.5797, -76.8875) -> (-16.0231, -79.3875)
  line L478 (-11.693, -76.8875) -> (-14.5797, -76.8875)
  line L479 (-10.2496, -79.3875) -> (-11.693, -76.8875)
  line L480 (-6.7443, -84.7447) -> (-5.3009, -82.2447)
  line L481 (-9.631, -84.7447) -> (-6.7443, -84.7447)
  line L482 (-11.0744, -82.2447) -> (-9.631, -84.7447)
  line L483 (-9.631, -79.7447) -> (-11.0744, -82.2447)
  line L484 (-6.7443, -79.7447) -> (-9.631, -79.7447)
  line L485 (-5.3009, -82.2447) -> (-6.7443, -79.7447)
  line L486 (-1.7956, -87.6018) -> (-0.3522, -85.1018)
  line L487 (-4.6823, -87.6018) -> (-1.7956, -87.6018)
  line L488 (-6.1257, -85.1018) -> (-4.6823, -87.6018)
  line L489 (-4.6823, -82.6018) -> (-6.1257, -85.1018)
  line L490 (-1.7956, -82.6018) -> (-4.6823, -82.6018)
  line L491 (-0.3522, -85.1018) -> (-1.7956, -82.6018)
  line L492 (3.1532, -90.459) -> (4.5965, -87.959)
  line L493 (0.2664, -90.459) -> (3.1532, -90.459)
  line L494 (-1.177, -87.959) -> (0.2664, -90.459)
  line L495 (0.2664, -85.459) -> (-1.177, -87.959)
  line L496 (3.1532, -85.459) -> (0.2664, -85.459)
  line L497 (4.5965, -87.959) -> (3.1532, -85.459)
  line L498 (8.1019, -93.3161) -> (9.5453, -90.8161)
  line L499 (5.2151, -93.3161) -> (8.1019, -93.3161)
  line L500 (3.7718, -90.8161) -> (5.2151, -93.3161)
  line L501 (5.2151, -88.3161) -> (3.7718, -90.8161)
  line L502 (8.1019, -88.3161) -> (5.2151, -88.3161)
  line L503 (9.5453, -90.8161) -> (8.1019, -88.3161)
  line L504 (13.0506, -96.1733) -> (14.494, -93.6733)
  line L505 (10.1638, -96.1733) -> (13.0506, -96.1733)
  line L506 (8.7205, -93.6733) -> (10.1638, -96.1733)
  line L507 (10.1638, -91.1733) -> (8.7205, -93.6733)
  line L508 (13.0506, -91.1733) -> (10.1638, -91.1733)
  line L509 (14.494, -93.6733) -> (13.0506, -91.1733)
  line L510 (17.9993, -99.0304) -> (19.4427, -96.5304)
  line L511 (15.1126, -99.0304) -> (17.9993, -99.0304)
  line L512 (13.6692, -96.5304) -> (15.1126, -99.0304)
  line L513 (15.1126, -94.0304) -> (13.6692, -96.5304)
  line L514 (17.9993, -94.0304) -> (15.1126, -94.0304)
  line L515 (19.4427, -96.5304) -> (17.9993, -94.0304)
  line L516 (22.948, -101.8875) -> (24.3914, -99.3875)
  line L517 (20.0613, -101.8875) -> (22.948, -101.8875)
  line L518 (18.6179, -99.3875) -> (20.0613, -101.8875)
  line L519 (20.0613, -96.8875) -> (18.6179, -99.3875)
  line L520 (22.948, -96.8875) -> (20.0613, -96.8875)
  line L521 (24.3914, -99.3875) -> (22.948, -96.8875)
  line L522 (27.8967, -104.7447) -> (29.3401, -102.2447)
  line L523 (25.01, -104.7447) -> (27.8967, -104.7447)
  line L524 (23.5666, -102.2447) -> (25.01, -104.7447)
  line L525 (25.01, -99.7447) -> (23.5666, -102.2447)
  line L526 (27.8967, -99.7447) -> (25.01, -99.7447)
  line L527 (29.3401, -102.2447) -> (27.8967, -99.7447)
  line L528 (32.8455, -107.6018) -> (34.2888, -105.1018)
  line L529 (29.9587, -107.6018) -> (32.8455, -107.6018)
  line L530 (28.5153, -105.1018) -> (29.9587, -107.6018)
  line L531 (29.9587, -102.6018) -> (28.5153, -105.1018)
  line L532 (32.8455, -102.6018) -> (29.9587, -102.6018)
  line L533 (34.2888, -105.1018) -> (32.8455, -102.6018)
  line L534 (37.7942, -110.459) -> (39.2376, -107.959)
  line L535 (34.9074, -110.459) -> (37.7942, -110.459)
  line L536 (33.4641, -107.959) -> (34.9074, -110.459)
  line L537 (34.9074, -105.459) -> (33.4641, -107.959)
  line L538 (37.7942, -105.459) -> (34.9074, -105.459)
  line L539 (39.2376, -107.959) -> (37.7942, -105.459)
  line L540 (42.7429, -113.3161) -> (44.1863, -110.8161)
  line L541 (39.8561, -113.3161) -> (42.7429, -113.3161)
  line L542 (38.4128, -110.8161) -> (39.8561, -113.3161)
  line L543 (39.8561, -108.3161) -> (38.4128, -110.8161)
  line L544 (42.7429, -108.3161) -> (39.8561, -108.3161)
  line L545 (44.1863, -110.8161) -> (42.7429, -108.3161)
  line L546 (47.6916, -116.1733) -> (49.135, -113.6733)
  line L547 (44.8049, -116.1733) -> (47.6916, -116.1733)
  line L548 (43.3615, -113.6733) -> (44.8049, -116.1733)
  line L549 (44.8049, -111.1733) -> (43.3615, -113.6733)
  line L550 (47.6916, -111.1733) -> (44.8049, -111.1733)
  line L551 (49.135, -113.6733) -> (47.6916, -111.1733)
  line L552 (52.6403, -119.0304) -> (54.0837, -116.5304)
  line L553 (49.7536, -119.0304) -> (52.6403, -119.0304)
  line L554 (48.3102, -116.5304) -> (49.7536, -119.0304)
  line L555 (49.7536, -114.0304) -> (48.3102, -116.5304)
  line L556 (52.6403, -114.0304) -> (49.7536, -114.0304)
  line L557 (54.0837, -116.5304) -> (52.6403, -114.0304)
  line L558 (-11.693, -76.1733) -> (-10.2496, -73.6733)
  line L559 (-14.5797, -76.1733) -> (-11.693, -76.1733)
  line L560 (-16.0231, -73.6733) -> (-14.5797, -76.1733)
  line L561 (-14.5797, -71.1733) -> (-16.0231, -73.6733)
  line L562 (-11.693, -71.1733) -> (-14.5797, -71.1733)
  line L563 (-10.2496, -73.6733) -> (-11.693, -71.1733)
  line L564 (-6.7443, -79.0304) -> (-5.3009, -76.5304)
  line L565 (-9.631, -79.0304) -> (-6.7443, -79.0304)
  line L566 (-11.0744, -76.5304) -> (-9.631, -79.0304)
  line L567 (-9.631, -74.0304) -> (-11.0744, -76.5304)
  line L568 (-6.7443, -74.0304) -> (-9.631, -74.0304)
  line L569 (-5.3009, -76.5304) -> (-6.7443, -74.0304)
  line L570 (-1.7956, -81.8875) -> (-0.3522, -79.3875)
  line L571 (-4.6823, -81.8875) -> (-1.7956, -81.8875)
  line L572 (-6.1257, -79.3875) -> (-4.6823, -81.8875)
  line L573 (-4.6823, -76.8875) -> (-6.1257, -79.3875)
  line L574 (-1.7956, -76.8875) -> (-4.6823, -76.8875)
  line L575 (-0.3522, -79.3875) -> (-1.7956, -76.8875)
  line L576 (3.1532, -84.7447) -> (4.5965, -82.2447)
  line L577 (0.2664, -84.7447) -> (3.1532, -84.7447)
  line L578 (-1.177, -82.2447) -> (0.2664, -84.7447)
  line L579 (0.2664, -79.7447) -> (-1.177, -82.2447)
  line L580 (3.1532, -79.7447) -> (0.2664, -79.7447)
  line L581 (4.5965, -82.2447) -> (3.1532, -79.7447)
  line L582 (8.1019, -87.6018) -> (9.5453, -85.1018)
  line L583 (5.2151, -87.6018) -> (8.1019, -87.6018)
  line L584 (3.7718, -85.1018) -> (5.2151, -87.6018)
  line L585 (5.2151, -82.6018) -> (3.7718, -85.1018)
  line L586 (8.1019, -82.6018) -> (5.2151, -82.6018)
  line L587 (9.5453, -85.1018) -> (8.1019, -82.6018)
  line L588 (13.0506, -90.459) -> (14.494, -87.959)
  line L589 (10.1638, -90.459) -> (13.0506, -90.459)
  line L590 (8.7205, -87.959) -> (10.1638, -90.459)
  line L591 (10.1638, -85.459) -> (8.7205, -87.959)
  line L592 (13.0506, -85.459) -> (10.1638, -85.459)
  line L593 (14.494, -87.959) -> (13.0506, -85.459)
  line L594 (17.9993, -93.3161) -> (19.4427, -90.8161)
  line L595 (15.1126, -93.3161) -> (17.9993, -93.3161)
  line L596 (13.6692, -90.8161) -> (15.1126, -93.3161)
  line L597 (15.1126, -88.3161) -> (13.6692, -90.8161)
  line L598 (17.9993, -88.3161) -> (15.1126, -88.3161)
  line L599 (19.4427, -90.8161) -> (17.9993, -88.3161)
  line L600 (22.948, -96.1733) -> (24.3914, -93.6733)
  line L601 (20.0613, -96.1733) -> (22.948, -96.1733)
  line L602 (18.6179, -93.6733) -> (20.0613, -96.1733)
  line L603 (20.0613, -91.1733) -> (18.6179, -93.6733)
  line L604 (22.948, -91.1733) -> (20.0613, -91.1733)
  line L605 (24.3914, -93.6733) -> (22.948, -91.1733)
  line L606 (27.8967, -99.0304) -> (29.3401, -96.5304)
  line L607 (25.01, -99.0304) -> (27.8967, -99.0304)
  line L608 (23.5666, -96.5304) -> (25.01, -99.0304)
  line L609 (25.01, -94.0304) -> (23.5666, -96.5304)
  line L610 (27.8967, -94.0304) -> (25.01, -94.0304)
  line L611 (29.3401, -96.5304) -> (27.8967, -94.0304)
  line L612 (32.8455, -101.8875) -> (34.2888, -99.3875)
  line L613 (29.9587, -101.8875) -> (32.8455, -101.8875)
  line L614 (28.5153, -99.3875) -> (29.9587, -101.8875)
  line L615 (29.9587, -96.8875) -> (28.5153, -99.3875)
  line L616 (32.8455, -96.8875) -> (29.9587, -96.8875)
  line L617 (34.2888, -99.3875) -> (32.8455, -96.8875)
  line L618 (37.7942, -104.7447) -> (39.2376, -102.2447)
  line L619 (34.9074, -104.7447) -> (37.7942, -104.7447)
  line L620 (33.4641, -102.2447) -> (34.9074, -104.7447)
  line L621 (34.9074, -99.7447) -> (33.4641, -102.2447)
  line L622 (37.7942, -99.7447) -> (34.9074, -99.7447)
  line L623 (39.2376, -102.2447) -> (37.7942, -99.7447)
  line L624 (42.7429, -107.6018) -> (44.1863, -105.1018)
  line L625 (39.8561, -107.6018) -> (42.7429, -107.6018)
  line L626 (38.4128, -105.1018) -> (39.8561, -107.6018)
  line L627 (39.8561, -102.6018) -> (38.4128, -105.1018)
  line L628 (42.7429, -102.6018) -> (39.8561, -102.6018)
  line L629 (44.1863, -105.1018) -> (42.7429, -102.6018)
  line L630 (47.6916, -110.459) -> (49.135, -107.959)
  line L631 (44.8049, -110.459) -> (47.6916, -110.459)
  line L632 (43.3615, -107.959) -> (44.8049, -110.459)
  line L633 (44.8049, -105.459) -> (43.3615, -107.959)
  line L634 (47.6916, -105.459) -> (44.8049, -105.459)
  line L635 (49.135, -107.959) -> (47.6916, -105.459)
  line L636 (52.6403, -113.3161) -> (54.0837, -110.8161)
  line L637 (49.7536, -113.3161) -> (52.6403, -113.3161)
  line L638 (48.3102, -110.8161) -> (49.7536, -113.3161)
  line L639 (49.7536, -108.3161) -> (48.3102, -110.8161)
  line L640 (52.6403, -108.3161) -> (49.7536, -108.3161)
  line L641 (54.0837, -110.8161) -> (52.6403, -108.3161)
  line L642 (57.589, -116.1733) -> (59.0324, -113.6733)
  line L643 (54.7023, -116.1733) -> (57.589, -116.1733)
  line L644 (53.2589, -113.6733) -> (54.7023, -116.1733)
  line L645 (54.7023, -111.1733) -> (53.2589, -113.6733)
  line L646 (57.589, -111.1733) -> (54.7023, -111.1733)
  line L647 (59.0324, -113.6733) -> (57.589, -111.1733)
  line L648 (-6.7443, -73.3161) -> (-5.3009, -70.8161)
  line L649 (-9.631, -73.3161) -> (-6.7443, -73.3161)
  line L650 (-11.0744, -70.8161) -> (-9.631, -73.3161)
  line L651 (-9.631, -68.3161) -> (-11.0744, -70.8161)